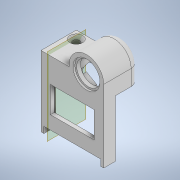
# Autodesk Inventor part: DeckelClip
Saved by Autodesk Inventor 2020.3 (Build 243373000, 373)
## iProperties
Created: 2020-05-20
Part Number: DeckelClip
Material: Generisch
Document SubType Name: Modeling
Designer: hpcwoess
Density: 1 g/cm^3
Appearance: Vorgabe
Author: hpcwoess
Autodesk Inventor part; units mm, degrees
ref_plane "YZ Plane" through (0, 0, 0) normal (1, 0, 0) x (0, 1, 0)
ref_plane "XZ Plane" through (0, 0, 0) normal (0, 1, 0) x (-1, 0, 0)
ref_plane "XY Plane" through (0, 0, 0) normal (0, 0, 1) x (1, 0, 0)
sketch "Skizze1" plane through (0, 0, 0) normal (0, 0, 1) x (1, 0, 0)
  line L0 (-16, 19.3) -> (-1.6, 19.3)
  line L1 (16, 20.3) -> (16, -16.7)
  line L2 (-16, -16.7) -> (-16, 19.3)
  line L3 (-11.2, 6.7) -> (11.2, 6.7)
  line L4 (11.2, 6.7) -> (11.2, -6.7)
  line L5 (11.2, -6.7) -> (-11.2, -6.7)
  line L6 (-11.2, -6.7) -> (-11.2, 6.7)
  circle A0 centre (7.2, 20.3) radius 6
  line L7 (16, -16.7) -> (-16, -16.7)
  line L8 (-1.6, 20.3) -> (-1.6, 19.3)
  arc A1 (16, 20.3) -> (-1.6, 20.3) centre (7.2, 20.3) ccw
  point P0 (0, 0)
  point P1 (5.2, -16.7)
  dimension "d0" = 22.4
  dimension "d1" = 11.2
  dimension "d3" = 16
  dimension "d4" = 13.4
  dimension "d5" = 6.7
  dimension "d32" = 12
  dimension "d43" = 36
  dimension "d62" = 16
  dimension "d68" = 8.8
  dimension "d69" = 8.8
  dimension "d72" = 37
  dimension "d73" = 0
  dimension "d82" = 10
  constraints: 18 end point, 4 parallel, 3 perpendicular, 2 centre point, 2 horizontal, 2 point on circle, 2 tangent, 1 point on line
  measures "d0" distance between parallel lines of L4 L6
  measures "d1" distance from line of L4 point (0, 0)
  measures "d3" distance from line of L2 point (0, 0)
  measures "d4" distance between parallel lines of L5 L3
  measures "d5" distance from line of L5 point (0, 0)
  measures "d32" diameter of A0
  measures "d43" distance between parallel lines of L7 L0
  measures "d62" distance from line of L1 point (0, 0)
  measures "d68" distance from line of L1 A0.centre
  measures "d69" radius of A1
  measures "d72" distance from line of A1.centre L7
  measures "d73" distance of A0.centre A1.centre
  measures "d82" distance between parallel lines of L5 L7
extrude "Extrusion1" add sketch "Skizze1" along normal blind 6
sketch "Skizze2" plane through (0, 0, 0) normal (0, 0, -1) x (-1, 0, 0)
  line L0 (-12.7, 7.3) -> (12.7, 7.3)
  line L1 (12.7, 7.3) -> (12.7, -10.3)
  line L2 (12.7, -10.3) -> (-12.7, -10.3)
  line L3 (-12.7, -10.3) -> (-12.7, 7.3)
  line L4 (11.2, 6.7) -> (-11.2, 6.7) projected
  line L5 (-4.5, -10.3) -> (4.5, -10.3)
  line L6 (4.5, -10.3) -> (4.5, -15.2)
  line L7 (4.5, -15.2) -> (-4.5, -15.2)
  line L8 (-4.5, -15.2) -> (-4.5, -10.3)
  line L9 (-6, 12.1) -> (6, 12.1)
  line L10 (6, 12.1) -> (6, 9.3)
  line L11 (6, 9.3) -> (-6, 9.3)
  line L12 (-6, 9.3) -> (-6, 12.1)
  line L13 (16, -16.7) -> (-16, -16.7) projected
  point P0 (0, 0)
  point P1 (4.5, -10.3)
  point P2 (-5.2, -16.5)
  point P3 (-16, -16.7)
  dimension "d11" = 25.4
  dimension "d12" = 17.6
  dimension "d24" = 9
  dimension "d25" = 4.5
  dimension "d26" = 12
  dimension "d27" = 6
  dimension "d28" = 2.8
  dimension "d29" = 2
  dimension "d44" = 6.4
  dimension "d45" = 12.7
  dimension "d46" = 4.9
  constraints: 24 end point, 6 parallel, 3 horizontal, 3 perpendicular, 1 point on line, 1 other
  measures "d11" distance of L0.start L0.end
  measures "d12" distance of L0.end L1.end
  measures "d24" distance between parallel lines of L8 L6
  measures "d25" distance from line of L6 point (0, 0)
  measures "d26" distance between parallel lines of L10 L12
  measures "d27" distance from line of L10 point (0, 0)
  measures "d28" distance between parallel lines of L9 L11
  measures "d29" distance between parallel lines of L0 L11
  measures "d45" distance from line of L1 point (0, 0)
  measures "d46" distance between parallel lines of L5 L7
extrude "Extrusion2" cut sketch "Skizze2" against normal blind 4
sketch "Skizze3" plane through (0, 0, 0) normal (0, 0, -1) x (-1, 0, 0)
  line L0 (-14.5, 12.3) -> (14.5, 12.3)
  line L1 (14.5, 12.3) -> (14.5, -15.5)
  line L2 (14.5, -15.5) -> (-14.5, -15.5)
  line L3 (-14.5, -15.5) -> (-14.5, 12.3)
  line L4 (16, 20.3) -> (16, -16.7) projected
  line L5 (-16, -16.7) -> (-16, 20.3) projected
  line L6 (16, -16.7) -> (-16, -16.7) projected
  point P0 (0, 0)
  point P1 (-15.2, -22)
  point P2 (-14.5619, 17.7435)
  point P3 (-5.2, -16.5)
  point P4 (-15.2, 17)
  dimension "d19" = 1.5
  dimension "d20" = 1.5
  dimension "d54" = 1.2
  dimension "d55" = 27.8
  constraints: 8 end point, 2 parallel, 1 horizontal, 1 perpendicular, 3 other
  measures "d55" distance between parallel lines of L2 L0
extrude "Extrusion3" cut sketch "Skizze3" against normal blind 2.2
sketch "Skizze5" plane through (0, 0, 0) normal (0, 0, -1) x (-1, 0, 0)
  circle A0 centre (-7.2, 20.3) radius 6 projected
  circle A1 centre (-7.2, 20.3) radius 8.1
  line L0 (-0.7, 15.7389) -> (-6.5, 12.3903)
  line L1 (-7.9, 12.3903) -> (-13.7, 15.7389)
  line L2 (-14.4, 16.9514) -> (-14.4, 23.6486)
  line L3 (-13.7, 24.8611) -> (-7.9, 28.2097)
  line L4 (-6.5, 28.2097) -> (-0.7, 24.8611)
  line L5 (0, 23.6486) -> (0, 16.9514)
  arc A2 (0, 23.6486) -> (-0.7, 24.8611) centre (-1.4, 23.6486) ccw
  arc A3 (-0.7, 15.7389) -> (0, 16.9514) centre (-1.4, 16.9514) ccw
  arc A4 (-6.5, 28.2097) -> (-7.9, 28.2097) centre (-7.2, 26.9973) ccw
  arc A5 (-7.9, 12.3903) -> (-6.5, 12.3903) centre (-7.2, 13.6027) ccw
  arc A6 (-14.4, 16.9514) -> (-13.7, 15.7389) centre (-13, 16.9514) ccw
  arc A7 (-13.7, 24.8611) -> (-14.4, 23.6486) centre (-13, 23.6486) ccw
  point P0 (0, 0)
  point P1 (0, 16.1431)
  point P2 (-7.2, 11.9862)
  point P3 (-14.4, 16.1431)
  point P4 (-14.4, 24.4569)
  point P5 (-7.2, 28.6138)
  point P6 (0, 24.4569)
  dimension "d51" = 16.2
  dimension "d74" = 14.4
  dimension "d75" = 1.4
  dimension "d76" = 1.4
  dimension "d77" = 1.4
  constraints: 12 end point, 12 point on circle, 12 point on line, 12 tangent, 7 centre point, 3 equal radius, 2 coincident, 1 vertical, 13 other
  measures "d51" diameter of A1
  measures "d74" distance between parallel lines of L1 L4
  measures "d75" radius of A2
  measures "d76" radius of A3
  measures "d77" radius of A4
extrude "Extrusion5" cut sketch "Skizze5" against normal blind 3 contours L0 A5 L1 A6 L2 A7 L3 A4 L4 A2 L5 A3
sketch "Skizze7" plane through (0, 0, 6) normal (0, 0, 1) x (1, 0, 0)
  circle A0 centre (7.2, 20.3) radius 6 projected
  circle A1 centre (7.2, 20.3) radius 6.9
  point P0 (0, 0)
  dimension "d58" = 13.8
  constraints: 1 centre point, 1 coincident
  measures "d58" diameter of A1
extrude "Extrusion7" cut sketch "Skizze7" against normal blind 1 contours A0 | A1
sketch "Skizze8" plane through (0, 0, 0) normal (0, 0, -1) x (-1, 0, 0)
  arc A0 (-7.9, 12.3903) -> (-7.7127, 12.3) centre (-7.2, 13.6027) ccw projected
  line L0 (-7.9, 12.3903) -> (-13.7, 15.7389) projected
  arc A1 (-14.4, 16.9514) -> (-13.7, 15.7389) centre (-13, 16.9514) ccw projected
  line L1 (-14.4, 16.9514) -> (-14.4, 23.6486) projected
  arc A2 (-13.7, 24.8611) -> (-14.4, 23.6486) centre (-13, 23.6486) ccw projected
  line L2 (-13.7, 24.8611) -> (-7.9, 28.2097) projected
  arc A3 (-6.5, 28.2097) -> (-7.9, 28.2097) centre (-7.2, 26.9973) ccw projected
  line L3 (-6.5, 28.2097) -> (-0.7, 24.8611) projected
  arc A4 (0, 23.6486) -> (-0.7, 24.8611) centre (-1.4, 23.6486) ccw projected
  line L4 (0, 23.6486) -> (0, 16.9514) projected
  arc A5 (-0.7, 15.7389) -> (0, 16.9514) centre (-1.4, 16.9514) ccw projected
  line L5 (-0.7, 15.7389) -> (-6.5, 12.3903) projected
  arc A6 (-6.6873, 12.3) -> (-6.5, 12.3903) centre (-7.2, 13.6027) ccw projected
  line L6 (-6.6873, 12.3) -> (14.5, 12.3) projected
  line L7 (14.5, 12.3) -> (14.5, -15.5) projected
  line L8 (14.5, -15.5) -> (-14.5, -15.5) projected
  line L9 (-14.5, -15.5) -> (-14.5, 12.3) projected
  line L10 (-14.5, 12.3) -> (-7.7127, 12.3) projected
  line L11 (16, 19.3) -> (16, -16.7) projected
  line L12 (1.6, 19.3) -> (16, 19.3) projected
  line L13 (1.6, 20.3) -> (1.6, 19.3) projected
  arc A7 (1.6, 20.3) -> (-16, 20.3) centre (-7.2, 20.3) ccw projected
  line L14 (-16, -16.7) -> (-16, 20.3) projected
  line L15 (16, -16.7) -> (-16, -16.7) projected
  line L16 (-14.4, 16.9514) -> (-14.4, 12.3)
  line L17 (-14.5, 12.3) -> (-7.7127, 12.3) projected
  arc A8 (-0.7, 15.7389) -> (0, 16.9514) centre (-1.4, 16.9514) ccw projected
  line L18 (0, 16.9514) -> (0, 12.3)
  line L19 (-14.5, -15.5) -> (-14.5, 12.3) projected
  line L20 (-14.5, 12.3) -> (-16, 12.3)
  line L21 (0, 12.3) -> (16, 12.3)
  point P0 (0, 0)
  constraints: 8 end point, 5 point on line, 3 perpendicular, 1 tangent
extrude "Extrusion8" add sketch "Skizze8" along normal blind 3 contours L10 L20 L14 A7 L13 L12 L11 L21 L6 L18 L4 A4 L3 A3 L2 A2 L1 L16
sketch "Skizze9" plane through (0, 0, -3) normal (0, 0, -1) x (-1, 0, 0)
  arc A0 (-13.7, 24.8611) -> (-14.4, 23.6486) centre (-13, 23.6486) ccw projected
  line L0 (-13.7, 24.8611) -> (-7.9, 28.2097) projected
  arc A1 (-6.5, 28.2097) -> (-7.9, 28.2097) centre (-7.2, 26.9973) ccw projected
  line L1 (-6.5, 28.2097) -> (-0.7, 24.8611) projected
  arc A2 (0, 23.6486) -> (-0.7, 24.8611) centre (-1.4, 23.6486) ccw projected
  line L2 (0, 23.6486) -> (0, 12.3) projected
  line L3 (0, 12.3) -> (16, 12.3) projected
  line L4 (16, 12.3) -> (16, 19.3) projected
  line L5 (16, 19.3) -> (1.6, 19.3) projected
  line L6 (1.6, 19.3) -> (1.6, 20.3) projected
  arc A3 (1.6, 20.3) -> (-16, 20.3) centre (-7.2, 20.3) ccw projected
  line L7 (-16, 20.3) -> (-16, 12.3) projected
  line L8 (-16, 12.3) -> (-14.4, 12.3) projected
  line L9 (-14.4, 12.3) -> (-14.4, 23.6486) projected
  circle A4 centre (-7.2, 20.3) radius 6 projected
  line L10 (-13.2, 20.3) -> (-13.2, 12.3)
  line L11 (-14.5, 12.3) -> (-7.7127, 12.3) projected
  line L12 (-13.2, 12.3) -> (-14.5, 12.3)
  line L13 (-1.2, 20.3) -> (-1.2, 12.3)
  line L14 (-1.2, 12.3) -> (0, 12.3)
  line L15 (0, 12.3) -> (16, 12.3) projected
  point P0 (0, 0)
  constraints: 8 end point, 2 perpendicular, 2 point on circle, 1 collinear
extrude "Extrusion9" add sketch "Skizze9" along normal blind 7 contours L0 A1 L1 A2 L2 L14 L13 A4 L10 L11 L9 A0 | A0 L9 L8 L7 A3 L6 L5 L4 L3 L2 A2 L1 A1 L0
sketch "Skizze10" plane through (0, 0, -10) normal (0, 0, -1) x (-1, 0, 0)
  line L0 (-13.2, 12.3) -> (-13.2, 20.3) projected
  arc A0 (-1.2, 20.3) -> (-13.2, 20.3) centre (-7.2, 20.3) ccw projected
  line L1 (-1.2, 20.3) -> (-1.2, 12.3) projected
  line L2 (-1.2, 12.3) -> (16, 12.3) projected
  line L3 (16, 12.3) -> (16, 19.3) projected
  line L4 (16, 19.3) -> (1.6, 19.3) projected
  line L5 (1.6, 19.3) -> (1.6, 20.3) projected
  arc A1 (1.6, 20.3) -> (-16, 20.3) centre (-7.2, 20.3) ccw projected
  line L6 (-16, 20.3) -> (-16, 12.3) projected
  line L7 (-16, 12.3) -> (-13.2, 12.3) projected
  line L8 (-1.2, 12.3) -> (-13.2, 12.3)
  line L9 (-14.5, 12.3) -> (-7.7127, 12.3) projected
  point P0 (0, 0)
  constraints: 2 end point, 1 collinear
extrude "Extrusion10" add sketch "Skizze10" along normal blind 2
fillet "Rundung3" radius 2 3 edges at (7.2, 26.3, -10) (13.2, 16.3, -10) (1.2, 16.3, -10)
fillet "Rundung4" radius 4 3 edges at (7.2, 29.1, -12) (16, 16.3, -12) (-1.6, 19.8, -12)
sketch "Skizze11" plane through (-16, -16.7, 6) normal (-1, 0, 0) x (0, 0, 1)
  line L0 (-6, 29) -> (-18, 29) projected
  circle A0 centre (-9, 29) radius 2
  line L1 (-6, 29) -> (-6, 0) projected
  point P0 (-6, 16.7)
  point P1 (-11, 29)
  point P2 (-7, 29)
  dimension "d87" = 4
  dimension "d88" = 3
  constraints: 1 centre point, 1 point on line
  measures "d87" diameter of A0
  measures "d88" distance from line of A0.centre L1
extrude "Extrusion11" cut sketch "Skizze11" against normal blind 20.25 contours L0 A0 picked at (-8.7636, 29.6233)
sketch "Skizze12" plane through (-16, 19.3, 6) normal (0, 1, 0) x (1, 0, 0)
  circle A0 centre (4, 14) radius 1.75
  line L0 (0, 18) -> (0, 0) projected
  line L1 (0, 18) -> (18.4, 18) projected
  point P0 (16, 6)
  dimension "d91" = 3.5
  dimension "d92" = 4
  dimension "d93" = 4
  constraints: 1 centre point
  measures "d91" diameter of A0
  measures "d92" distance from line of L0 A0.centre
  measures "d93" distance from line of L1 A0.centre
extrude "Extrusion12" cut sketch "Skizze12" against normal blind 10
sketch "Skizze13" plane through (1.2, 12.3, -8) normal (1, 0, 0) x (0, 0, -1)
  circle A0 centre (-5.2, -0.0114) radius 5.5
  line L0 (-10.2, 0) -> (-10.2, -27.8) projected
  point P0 (-8, -12.3)
  dimension "d96" = 5
  dimension "d97" = 11
  constraints: 1 centre point
  measures "d96" distance from line of A0.centre L0
  measures "d97" diameter of A0
extrude "Extrusion13" cut sketch "Skizze13" against normal blind 10
ref_plane "Arbeitsebene1" through (-12, -16.7, 6) normal (-1, 0, 0) x (0, 0, 1)
sketch "Skizze14" plane through (-12, -16.7, 6) normal (-1, 0, 0) x (0, 0, 1)
  arc A0 (-7, 29) -> (-11, 29) centre (-9, 29) ccw projected
  arc A1 (-7.1, 29) -> (-10.9, 29) centre (-9, 29) ccw
  line L0 (-7, 29) -> (-7.1, 29)
  line L1 (-6, 29) -> (-14, 29) projected
  line L2 (-11, 29) -> (-10.9, 29)
  point P0 (-6, 16.7)
  dimension "d101" = 1.9
  constraints: 4 end point, 3 point on line, 2 point on circle, 1 centre point, 1 coincident
  measures "d101" radius of A1
extrude "Extrusion14" add sketch "Skizze14" along normal mid plane 0.5 contours L0 A1 L1 A0
chamfer "Fase1" distance 1.5 angle 45 1 edges at (-13.75, 19.3, -8)
sketch "Skizze15" plane through (14.5, -15.5, 0) normal (-1, 0, 0) x (0, 0, 1)
  line L0 (0, 0) -> (2.2, 0) projected
  line L1 (0, 0) -> (4, 0)
  line L2 (4, 0) -> (4, 2)
  line L3 (0, -1.2) -> (6, -1.2) projected
  line L4 (6, -1.2) -> (6, 35.8) projected
  line L5 (4, 2) -> (6, 2)
  line L6 (0, -1.2) -> (0, 27.8) projected
  line L7 (0, 0) -> (0, -1.2)
  line L8 (0, -1.2) -> (6, -1.2)
  point P0 (0, 15.5)
  dimension "d107" = 2
  dimension "d108" = 2
  constraints: 10 end point, 2 horizontal, 2 perpendicular, 1 collinear, 1 point on line
  measures "d107" distance between parallel lines of L2 L4
  measures "d108" distance between parallel lines of L1 L5
extrude "Extrusion15" cut sketch "Skizze15" along normal up to surface (29 mm away)
equation "\"d1\" = 0.5 * d0"
equation "\"d3\" = d62"
equation "\"d5\" = 0.5 * d4"
equation "\"d68\" = d69"
equation "\"d25\" = 0.5 * d24"
equation "\"d27\" = 0.5 * d26"
equation "\"d45\" = 0.5 * d11"
equation "\"d93\" = d92"
equation "\"d42\" = d37"
equation "\"d37\" = 3.5"
